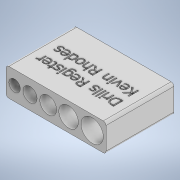
# Autodesk Inventor part: drillRegisterForKevin
Saved by Autodesk Inventor 2022.2 (Build 262287030, 287C)
## iProperties
Created: 2022-02-01
Part Number: drillRegisterForKevin
Material: Generic
Document SubType Name: Modeling
Designer: snobo
Density: 1 g/cm^3
Appearance: Default
Author: snobo
Autodesk Inventor part; units mm, degrees
ref_plane "YZ Plane" through (0, 0, 0) normal (1, 0, 0) x (0, 1, 0)
ref_plane "XZ Plane" through (0, 0, 0) normal (0, 1, 0) x (-1, 0, 0)
ref_plane "XY Plane" through (0, 0, 0) normal (0, 0, 1) x (1, 0, 0)
sketch "Sketch1" plane through (0, 0, 0) normal (0, 0, 1) x (1, 0, 0)
  circle A0 centre (0, 0) radius 13.0175
  circle A1 centre (-27.6225, 0) radius 11.43
  circle A2 centre (-51.4604, 0) radius 9.8425
  circle A3 centre (-72.7329, 0) radius 8.255
  circle A4 centre (-90.8304, 0) radius 6.6675
  line L0 (-90.8304, 0) -> (0, 0) construction
  line L1 (-100.6729, 16.1925) -> (16.1925, 16.1925)
  line L2 (16.1925, 16.1925) -> (16.1925, -16.1925)
  line L3 (16.1925, -16.1925) -> (-100.6729, -16.1925)
  line L4 (-100.6729, -16.1925) -> (-100.6729, 16.1925)
  dimension "d0" = 26.035
  dimension "d1" = 22.86
  dimension "d2" = 3.175
  dimension "d3" = 19.685
  dimension "d4" = 2.5654
  dimension "d5" = 3.175
  dimension "d6" = 16.51
  dimension "d7" = 3.175
  dimension "d8" = 13.335
  dimension "d9" = 3.175
  dimension "d10" = 3.175
  dimension "d11" = 3.175
  dimension "d12" = 3.175
  constraints: 10 end point, 5 centre point, 2 horizontal, 2 parallel, 1 coincident, 1 perpendicular
  measures "d0" diameter of A0
  measures "d1" diameter of A1
  measures "d3" diameter of A2
  measures "d6" diameter of A3
  measures "d8" diameter of A4
  measures "d9" distance edge to line of A0 L2
  measures "d10" distance edge to line of A4 L4
  measures "d11" distance edge to line of A0 L1
  measures "d12" distance edge to line of A0 L3
extrude "Extrusion1" add sketch "Sketch1" against normal blind 76.2
sketch "Sketch2" plane through (0, 0, -76.2) normal (0, 0, -1) x (-1, 0, 0)
  line L0 (-16.1925, -16.1925) -> (-16.1925, 16.1925) projected
  line L1 (-16.1925, 16.1925) -> (100.6729, 16.1925) projected
  line L2 (-16.1925, -16.1925) -> (100.6729, -16.1925)
  line L3 (100.6729, -16.1925) -> (100.6729, 16.1925)
  line L4 (100.6729, 16.1925) -> (-16.1925, 16.1925)
  line L5 (-16.1925, 16.1925) -> (-16.1925, -16.1925)
  point P0 (0, 0)
  constraints: 8 end point, 2 parallel, 1 horizontal, 1 perpendicular
extrude "Extrusion2" add sketch "Sketch2" along normal blind 3.175
fillet "Fillet1" radius 3.175 4 edges at (16.1925, 16.1925, -39.6875) (16.1925, -16.1925, -39.6875) (-100.6729, -16.1925, -39.6875) (-100.6729, 16.1925, -39.6875)
sketch "Sketch3" plane through (-97.4979, 16.1925, 0) normal (0, 1, 0) x (1, 0, 0)
  line L0 (0, 79.375) -> (0, 0) construction
  line L1 (0, 39.6875) -> (110.5154, 39.6875) construction
  line L2 (110.5154, 0) -> (110.5154, 79.375) construction
  spline S0 degree 2 poles (92.8637, 26.3618) (92.8637, 27.9271) (94.1327, 30.4466) (95.1979, 31.1505) knots 0 0 0 1 2 2 2
  spline S1 degree 2 poles (95.1979, 31.1505) (96.0685, 31.697) (97.8562, 32.0675) (99.2456, 32.0675) knots 0 0 0 1 2 2 2
  line L3 (99.2456, 32.0675) -> (101.8762, 32.0675)
  line L4 (101.8762, 32.0675) -> (101.8762, 20.6375)
  line L5 (101.8762, 20.6375) -> (99.2734, 20.6375)
  spline S2 degree 2 poles (99.2734, 20.6375) (97.6617, 20.6375) (95.8277, 21.1192) (95.1793, 21.5452) knots 0 0 0 1 2 2 2
  spline S3 degree 2 poles (95.1793, 21.5452) (94.0771, 22.277) (92.8637, 24.6945) (92.8637, 26.3618) knots 0 0 0 1 2 2 2
  spline S4 degree 2 poles (94.4476, 26.3432) (94.4476, 25.028) (95.3183, 23.1662) (96.1797, 22.6382) knots 0 0 0 1 2 2 2
  spline S5 degree 2 poles (96.1797, 22.6382) (96.791, 22.277) (98.1711, 21.9528) (99.1993, 21.9528) knots 0 0 0 1 2 2 2
  line L6 (99.1993, 21.9528) -> (100.3571, 21.9528)
  line L7 (100.3571, 21.9528) -> (100.3571, 30.7522)
  line L8 (100.3571, 30.7522) -> (99.1993, 30.7522)
  spline S6 degree 2 poles (99.1993, 30.7522) (98.1897, 30.7522) (96.6613, 30.428) (96.0408, 29.9927) knots 0 0 0 1 2 2 2
  spline S7 degree 2 poles (96.0408, 29.9927) (95.2442, 29.4555) (94.4476, 27.677) (94.4476, 26.3432) knots 0 0 0 1 2 2 2
  line L9 (86.7782, 25.0372) -> (86.8523, 25.0372)
  spline S8 degree 2 poles (86.8523, 25.0372) (87.019, 24.9909) (87.3803, 24.9724) (87.6304, 24.9724) knots 0 0 0 1 2 2 2
  spline S9 degree 2 poles (87.6304, 24.9724) (88.2139, 24.9724) (89.3624, 25.4818) (89.8812, 25.982) knots 0 0 0 1 2 2 2
  line L10 (89.8812, 25.982) -> (89.8812, 32.0675)
  line L11 (89.8812, 32.0675) -> (91.3261, 32.0675)
  line L12 (91.3261, 32.0675) -> (91.3261, 23.4904)
  line L13 (91.3261, 23.4904) -> (89.8812, 23.4904)
  line L14 (89.8812, 23.4904) -> (89.8812, 24.7686)
  spline S10 degree 2 poles (89.8812, 24.7686) (89.0938, 24.0646) (87.9175, 23.4904) (87.3617, 23.4904) knots 0 0 0 1 2 2 2
  spline S11 degree 2 poles (87.3617, 23.4904) (87.1394, 23.4904) (86.9171, 23.5089) (86.7782, 23.5367) knots 0 0 0 1 2 2 2
  line L15 (86.7782, 23.5367) -> (86.7782, 25.0372)
  line L16 (84.1847, 32.0675) -> (85.6296, 32.0675)
  line L17 (85.6296, 32.0675) -> (85.6296, 23.4904)
  line L18 (85.6296, 23.4904) -> (84.1847, 23.4904)
  line L19 (84.1847, 23.4904) -> (84.1847, 32.0675)
  line L20 (84.0828, 22.0639) -> (85.7223, 22.0639)
  line L21 (85.7223, 22.0639) -> (85.7223, 20.5634)
  line L22 (85.7223, 20.5634) -> (84.0828, 20.5634)
  line L23 (84.0828, 20.5634) -> (84.0828, 22.0639)
  line L24 (80.5908, 32.0675) -> (82.0358, 32.0675)
  line L25 (82.0358, 32.0675) -> (82.0358, 20.1281)
  line L26 (82.0358, 20.1281) -> (80.5908, 20.1281)
  line L27 (80.5908, 20.1281) -> (80.5908, 32.0675)
  line L28 (76.9969, 32.0675) -> (78.4419, 32.0675)
  line L29 (78.4419, 32.0675) -> (78.4419, 20.1281)
  line L30 (78.4419, 20.1281) -> (76.9969, 20.1281)
  line L31 (76.9969, 20.1281) -> (76.9969, 32.0675)
  spline S12 degree 2 poles (72.5602, 32.2713) (73.4216, 32.2713) (74.9129, 31.8081) (75.4038, 31.5488) knots 0 0 0 1 2 2 2
  line L32 (75.4038, 31.5488) -> (75.4038, 29.9278)
  line L33 (75.4038, 29.9278) -> (75.3297, 29.9278)
  spline S13 degree 2 poles (75.3297, 29.9278) (75.1444, 30.076) (74.6442, 30.428) (74.2274, 30.6225) knots 0 0 0 1 2 2 2
  spline S14 degree 2 poles (74.2274, 30.6225) (73.8662, 30.7985) (72.977, 31.0579) (72.5046, 31.0579) knots 0 0 0 1 2 2 2
  spline S15 degree 2 poles (72.5046, 31.0579) (72.1619, 31.0579) (71.3746, 30.9004) (71.1893, 30.7707) knots 0 0 0 1 2 2 2
  spline S16 degree 2 poles (71.1893, 30.7707) (70.9207, 30.5948) (70.6799, 30.1965) (70.6799, 29.7889) knots 0 0 0 1 2 2 2
  spline S17 degree 2 poles (70.6799, 29.7889) (70.6799, 29.2795) (71.2356, 28.7515) (71.9488, 28.5755) knots 0 0 0 1 2 2 2
  spline S18 degree 2 poles (71.9488, 28.5755) (72.2267, 28.5107) (73.1159, 28.3254) (73.4957, 28.2235) knots 0 0 0 1 2 2 2
  spline S19 degree 2 poles (73.4957, 28.2235) (74.4775, 27.9364) (75.3667, 26.7508) (75.3667, 25.9079) knots 0 0 0 1 2 2 2
  spline S20 degree 2 poles (75.3667, 25.9079) (75.3667, 24.7408) (73.6161, 23.2866) (72.1711, 23.2866) knots 0 0 0 1 2 2 2
  spline S21 degree 2 poles (72.1711, 23.2866) (71.4579, 23.2866) (70.013, 23.6386) (69.522, 23.9072) knots 0 0 0 1 2 2 2
  line L34 (69.522, 23.9072) -> (69.522, 25.454)
  line L35 (69.522, 25.454) -> (69.5961, 25.454)
  spline S22 degree 2 poles (69.5961, 25.454) (70.1519, 25.0094) (71.5042, 24.5) (72.1989, 24.5) knots 0 0 0 1 2 2 2
  spline S23 degree 2 poles (72.1989, 24.5) (72.9121, 24.5) (73.894, 25.1021) (73.894, 25.7041) knots 0 0 0 1 2 2 2
  spline S24 degree 2 poles (73.894, 25.7041) (73.894, 26.2506) (73.3104, 26.7786) (72.6621, 26.9453) knots 0 0 0 1 2 2 2
  spline S25 degree 2 poles (72.6621, 26.9453) (72.3471, 27.0287) (71.5505, 27.1954) (71.1152, 27.2973) knots 0 0 0 1 2 2 2
  spline S26 degree 2 poles (71.1152, 27.2973) (70.1704, 27.5381) (69.2071, 28.6404) (69.2071, 29.5944) knots 0 0 0 1 2 2 2
  spline S27 degree 2 poles (69.2071, 29.5944) (69.2071, 30.1501) (69.6425, 31.132) (70.0685, 31.4932) knots 0 0 0 1 2 2 2
  spline S28 degree 2 poles (70.0685, 31.4932) (70.5224, 31.873) (71.6802, 32.2713) (72.5602, 32.2713) knots 0 0 0 1 2 2 2
  line L36 (53.998, 32.0675) -> (55.9709, 32.0675)
  line L37 (55.9709, 32.0675) -> (59.5833, 27.5196)
  line L38 (59.5833, 27.5196) -> (61.3247, 27.5196)
  line L39 (61.3247, 27.5196) -> (61.3247, 32.0675)
  line L40 (61.3247, 32.0675) -> (62.8437, 32.0675)
  line L41 (62.8437, 32.0675) -> (62.8437, 20.6375)
  line L42 (62.8437, 20.6375) -> (59.8982, 20.6375)
  spline S29 degree 2 poles (59.8982, 20.6375) (58.9164, 20.6375) (57.5919, 20.8505) (56.9898, 21.2396) knots 0 0 0 1 2 2 2
  spline S30 degree 2 poles (56.9898, 21.2396) (56.3877, 21.6286) (55.693, 22.842) (55.693, 23.7405) knots 0 0 0 1 2 2 2
  spline S31 degree 2 poles (55.693, 23.7405) (55.693, 24.9909) (56.9713, 26.686) (58.0643, 27.0935) knots 0 0 0 1 2 2 2
  line L43 (58.0643, 27.0935) -> (53.998, 32.0675)
  spline S32 degree 2 poles (57.2769, 23.8609) (57.2769, 23.3607) (57.6289, 22.5919) (57.9994, 22.3418) knots 0 0 0 1 2 2 2
  spline S33 degree 2 poles (57.9994, 22.3418) (58.3236, 22.1288) (59.185, 21.9528) (59.8149, 21.9528) knots 0 0 0 1 2 2 2
  line L44 (59.8149, 21.9528) -> (61.3247, 21.9528)
  line L45 (61.3247, 21.9528) -> (61.3247, 26.2506)
  line L46 (61.3247, 26.2506) -> (59.9909, 26.2506)
  spline S34 degree 2 poles (59.9909, 26.2506) (59.3332, 26.2506) (58.2866, 26.019) (57.9253, 25.6578) knots 0 0 0 1 2 2 2
  spline S35 degree 2 poles (57.9253, 25.6578) (57.5919, 25.3429) (57.2769, 24.4537) (57.2769, 23.8609) knots 0 0 0 1 2 2 2
  spline S36 degree 2 poles (49.4779, 32.262) (51.5342, 32.262) (53.7942, 29.9556) (53.7942, 27.8252) knots 0 0 0 1 2 2 2
  spline S37 degree 2 poles (53.7942, 27.8252) (53.7942, 25.7319) (51.599, 23.2495) (49.8298, 23.2495) knots 0 0 0 1 2 2 2
  spline S38 degree 2 poles (49.8298, 23.2495) (49.0333, 23.2495) (47.8013, 23.7127) (47.3475, 24.2036) knots 0 0 0 1 2 2 2
  spline S39 degree 2 poles (47.3475, 24.2036) (46.8843, 24.6945) (46.3934, 26.1117) (46.3934, 27.1398) knots 0 0 0 1 2 2 2
  line L47 (46.3934, 27.1398) -> (46.3934, 27.9271)
  line L48 (46.3934, 27.9271) -> (52.3307, 27.9271)
  spline S40 degree 2 poles (52.3307, 27.9271) (52.3307, 29.4184) (50.8302, 31.0023) (49.4964, 31.0023) knots 0 0 0 1 2 2 2
  spline S41 degree 2 poles (49.4964, 31.0023) (49.024, 31.0023) (48.107, 30.7893) (47.7365, 30.6225) knots 0 0 0 1 2 2 2
  spline S42 degree 2 poles (47.7365, 30.6225) (47.3475, 30.4373) (46.8102, 30.1131) (46.6343, 29.9649) knots 0 0 0 1 2 2 2
  line L49 (46.6343, 29.9649) -> (46.5509, 29.9649)
  line L50 (46.5509, 29.9649) -> (46.5509, 31.5395)
  spline S43 degree 2 poles (46.5509, 31.5395) (46.801, 31.6414) (47.5605, 31.9378) (47.8569, 32.0212) knots 0 0 0 1 2 2 2
  spline S44 degree 2 poles (47.8569, 32.0212) (48.2737, 32.1416) (48.9592, 32.262) (49.4779, 32.262) knots 0 0 0 1 2 2 2
  spline S45 degree 2 poles (47.8013, 26.8249) (47.8199, 26.2413) (48.0607, 25.3892) (48.2923, 25.1021) knots 0 0 0 1 2 2 2
  spline S46 degree 2 poles (48.2923, 25.1021) (48.5423, 24.7779) (49.3297, 24.4351) (49.9132, 24.4351) knots 0 0 0 1 2 2 2
  spline S47 degree 2 poles (49.9132, 24.4351) (50.4875, 24.4351) (51.2933, 24.7779) (51.6268, 25.1113) knots 0 0 0 1 2 2 2
  spline S48 degree 2 poles (51.6268, 25.1113) (51.951, 25.454) (52.2844, 26.2784) (52.3307, 26.8249) knots 0 0 0 1 2 2 2
  line L51 (52.3307, 26.8249) -> (47.8013, 26.8249)
  spline S49 degree 2 poles (44.6243, 33.4384) (44.4761, 33.5032) (43.9111, 33.707) (43.5498, 33.7903) knots 0 0 0 1 2 2 2
  spline S50 degree 2 poles (43.5498, 33.7903) (43.1515, 33.8922) (42.4754, 34.0126) (42.0771, 34.0126) knots 0 0 0 1 2 2 2
  spline S51 degree 2 poles (42.0771, 34.0126) (41.4102, 34.0126) (40.4839, 33.6607) (40.2246, 33.3457) knots 0 0 0 1 2 2 2
  spline S52 degree 2 poles (40.2246, 33.3457) (39.9745, 33.0308) (39.78, 32.2064) (39.78, 31.6785) knots 0 0 0 1 2 2 2
  line L52 (39.78, 31.6785) -> (39.78, 30.9282)
  spline S53 degree 2 poles (39.78, 30.9282) (40.3635, 31.4376) (41.4843, 31.9193) (42.3272, 31.9193) knots 0 0 0 1 2 2 2
  spline S54 degree 2 poles (42.3272, 31.9193) (43.7907, 31.9193) (45.5227, 29.7426) (45.5227, 27.6956) knots 0 0 0 1 2 2 2
  spline S55 degree 2 poles (45.5227, 27.6956) (45.5227, 26.6304) (44.9207, 24.9816) (44.4205, 24.3981) knots 0 0 0 1 2 2 2
  spline S56 degree 2 poles (44.4205, 24.3981) (43.9389, 23.8516) (42.6143, 23.2495) (41.9104, 23.2495) knots 0 0 0 1 2 2 2
  spline S57 degree 2 poles (41.9104, 23.2495) (41.2434, 23.2495) (40.2709, 23.5645) (39.78, 23.8516) knots 0 0 0 1 2 2 2
  line L53 (39.78, 23.8516) -> (39.6966, 23.4904)
  line L54 (39.6966, 23.4904) -> (38.335, 23.4904)
  line L55 (38.335, 23.4904) -> (38.335, 31.0857)
  spline S58 degree 2 poles (38.335, 31.0857) (38.335, 33.2716) (40.2338, 35.3094) (42.1882, 35.3094) knots 0 0 0 1 2 2 2
  spline S59 degree 2 poles (42.1882, 35.3094) (42.8181, 35.3094) (44.1334, 35.1056) (44.6984, 34.9389) knots 0 0 0 1 2 2 2
  line L56 (44.6984, 34.9389) -> (44.6984, 33.4384)
  line L57 (44.6984, 33.4384) -> (44.6243, 33.4384)
  line L58 (39.78, 29.7426) -> (39.78, 25.028)
  spline S60 degree 2 poles (39.78, 25.028) (40.3172, 24.7686) (41.2249, 24.5463) (41.6788, 24.5463) knots 0 0 0 1 2 2 2
  spline S61 degree 2 poles (41.6788, 24.5463) (42.7718, 24.5463) (44.0315, 26.158) (44.0315, 27.6678) knots 0 0 0 1 2 2 2
  spline S62 degree 2 poles (44.0315, 27.6678) (44.0315, 29.0942) (43.0774, 30.5855) (42.003, 30.5855) knots 0 0 0 1 2 2 2
  spline S63 degree 2 poles (42.003, 30.5855) (41.438, 30.5855) (40.2524, 30.1409) (39.78, 29.7426) knots 0 0 0 1 2 2 2
  line L59 (34.7689, 32.0675) -> (36.2139, 32.0675)
  line L60 (36.2139, 32.0675) -> (36.2139, 23.4904)
  line L61 (36.2139, 23.4904) -> (34.7689, 23.4904)
  line L62 (34.7689, 23.4904) -> (34.7689, 32.0675)
  line L63 (34.667, 22.0639) -> (36.3065, 22.0639)
  line L64 (36.3065, 22.0639) -> (36.3065, 20.5634)
  line L65 (36.3065, 20.5634) -> (34.667, 20.5634)
  line L66 (34.667, 20.5634) -> (34.667, 22.0639)
  spline S64 degree 2 poles (30.3322, 32.2713) (31.1936, 32.2713) (32.6848, 31.8081) (33.1758, 31.5488) knots 0 0 0 1 2 2 2
  line L67 (33.1758, 31.5488) -> (33.1758, 29.9278)
  line L68 (33.1758, 29.9278) -> (33.1017, 29.9278)
  spline S65 degree 2 poles (33.1017, 29.9278) (32.9164, 30.076) (32.4162, 30.428) (31.9994, 30.6225) knots 0 0 0 1 2 2 2
  spline S66 degree 2 poles (31.9994, 30.6225) (31.6382, 30.7985) (30.749, 31.0579) (30.2766, 31.0579) knots 0 0 0 1 2 2 2
  spline S67 degree 2 poles (30.2766, 31.0579) (29.9339, 31.0579) (29.1465, 30.9004) (28.9613, 30.7707) knots 0 0 0 1 2 2 2
  spline S68 degree 2 poles (28.9613, 30.7707) (28.6927, 30.5948) (28.4519, 30.1965) (28.4519, 29.7889) knots 0 0 0 1 2 2 2
  spline S69 degree 2 poles (28.4519, 29.7889) (28.4519, 29.2795) (29.0076, 28.7515) (29.7208, 28.5755) knots 0 0 0 1 2 2 2
  spline S70 degree 2 poles (29.7208, 28.5755) (29.9987, 28.5107) (30.8879, 28.3254) (31.2677, 28.2235) knots 0 0 0 1 2 2 2
  spline S71 degree 2 poles (31.2677, 28.2235) (32.2495, 27.9364) (33.1387, 26.7508) (33.1387, 25.9079) knots 0 0 0 1 2 2 2
  spline S72 degree 2 poles (33.1387, 25.9079) (33.1387, 24.7408) (31.3881, 23.2866) (29.9431, 23.2866) knots 0 0 0 1 2 2 2
  spline S73 degree 2 poles (29.9431, 23.2866) (29.2299, 23.2866) (27.7849, 23.6386) (27.294, 23.9072) knots 0 0 0 1 2 2 2
  line L69 (27.294, 23.9072) -> (27.294, 25.454)
  line L70 (27.294, 25.454) -> (27.3681, 25.454)
  spline S74 degree 2 poles (27.3681, 25.454) (27.9239, 25.0094) (29.2762, 24.5) (29.9709, 24.5) knots 0 0 0 1 2 2 2
  spline S75 degree 2 poles (29.9709, 24.5) (30.6841, 24.5) (31.666, 25.1021) (31.666, 25.7041) knots 0 0 0 1 2 2 2
  spline S76 degree 2 poles (31.666, 25.7041) (31.666, 26.2506) (31.0824, 26.7786) (30.434, 26.9453) knots 0 0 0 1 2 2 2
  spline S77 degree 2 poles (30.434, 26.9453) (30.1191, 27.0287) (29.3225, 27.1954) (28.8872, 27.2973) knots 0 0 0 1 2 2 2
  spline S78 degree 2 poles (28.8872, 27.2973) (27.9424, 27.5381) (26.9791, 28.6404) (26.9791, 29.5944) knots 0 0 0 1 2 2 2
  spline S79 degree 2 poles (26.9791, 29.5944) (26.9791, 30.1501) (27.4144, 31.132) (27.8405, 31.4932) knots 0 0 0 1 2 2 2
  spline S80 degree 2 poles (27.8405, 31.4932) (28.2944, 31.873) (29.4522, 32.2713) (30.3322, 32.2713) knots 0 0 0 1 2 2 2
  spline S81 degree 2 poles (23.0425, 32.2342) (24.2189, 32.2342) (25.5434, 30.8912) (25.5434, 29.4369) knots 0 0 0 1 2 2 2
  line L71 (25.5434, 29.4369) -> (25.5434, 24.6852)
  line L72 (25.5434, 24.6852) -> (26.516, 24.6852)
  line L73 (26.516, 24.6852) -> (26.516, 23.4904)
  line L74 (26.516, 23.4904) -> (25.5434, 23.4904)
  line L75 (25.5434, 23.4904) -> (25.5434, 21.0265)
  line L76 (25.5434, 21.0265) -> (24.0984, 21.0265)
  line L77 (24.0984, 21.0265) -> (24.0984, 23.4904)
  line L78 (24.0984, 23.4904) -> (21.4401, 23.4904)
  line L79 (21.4401, 23.4904) -> (21.4401, 24.6852)
  line L80 (21.4401, 24.6852) -> (24.0984, 24.6852)
  line L81 (24.0984, 24.6852) -> (24.0984, 28.77)
  spline S82 degree 2 poles (24.0984, 28.77) (24.0984, 29.4184) (24.0521, 30.1316) (23.8947, 30.4373) knots 0 0 0 1 2 2 2
  spline S83 degree 2 poles (23.8947, 30.4373) (23.765, 30.7059) (23.1815, 30.9745) (22.6813, 30.9745) knots 0 0 0 1 2 2 2
  spline S84 degree 2 poles (22.6813, 30.9745) (22.3293, 30.9745) (21.6717, 30.7615) (21.5235, 30.6966) knots 0 0 0 1 2 2 2
  line L82 (21.5235, 30.6966) -> (21.4401, 30.6966)
  line L83 (21.4401, 30.6966) -> (21.4401, 31.9934)
  spline S85 degree 2 poles (21.4401, 31.9934) (21.8476, 32.1046) (22.6813, 32.2342) (23.0425, 32.2342) knots 0 0 0 1 2 2 2
  spline S86 degree 2 poles (16.6513, 32.262) (18.7076, 32.262) (20.9677, 29.9556) (20.9677, 27.8252) knots 0 0 0 1 2 2 2
  spline S87 degree 2 poles (20.9677, 27.8252) (20.9677, 25.7319) (18.7725, 23.2495) (17.0033, 23.2495) knots 0 0 0 1 2 2 2
  spline S88 degree 2 poles (17.0033, 23.2495) (16.2067, 23.2495) (14.9748, 23.7127) (14.521, 24.2036) knots 0 0 0 1 2 2 2
  spline S89 degree 2 poles (14.521, 24.2036) (14.0578, 24.6945) (13.5669, 26.1117) (13.5669, 27.1398) knots 0 0 0 1 2 2 2
  line L84 (13.5669, 27.1398) -> (13.5669, 27.9271)
  line L85 (13.5669, 27.9271) -> (19.5042, 27.9271)
  spline S90 degree 2 poles (19.5042, 27.9271) (19.5042, 29.4184) (18.0037, 31.0023) (16.6699, 31.0023) knots 0 0 0 1 2 2 2
  spline S91 degree 2 poles (16.6699, 31.0023) (16.1975, 31.0023) (15.2805, 30.7893) (14.91, 30.6225) knots 0 0 0 1 2 2 2
  spline S92 degree 2 poles (14.91, 30.6225) (14.521, 30.4373) (13.9837, 30.1131) (13.8077, 29.9649) knots 0 0 0 1 2 2 2
  line L86 (13.8077, 29.9649) -> (13.7244, 29.9649)
  line L87 (13.7244, 29.9649) -> (13.7244, 31.5395)
  spline S93 degree 2 poles (13.7244, 31.5395) (13.9745, 31.6414) (14.734, 31.9378) (15.0304, 32.0212) knots 0 0 0 1 2 2 2
  spline S94 degree 2 poles (15.0304, 32.0212) (15.4472, 32.1416) (16.1326, 32.262) (16.6513, 32.262) knots 0 0 0 1 2 2 2
  spline S95 degree 2 poles (14.9748, 26.8249) (14.9933, 26.2413) (15.2342, 25.3892) (15.4657, 25.1021) knots 0 0 0 1 2 2 2
  spline S96 degree 2 poles (15.4657, 25.1021) (15.7158, 24.7779) (16.5031, 24.4351) (17.0867, 24.4351) knots 0 0 0 1 2 2 2
  spline S97 degree 2 poles (17.0867, 24.4351) (17.661, 24.4351) (18.4668, 24.7779) (18.8003, 25.1113) knots 0 0 0 1 2 2 2
  spline S98 degree 2 poles (18.8003, 25.1113) (19.1245, 25.454) (19.4579, 26.2784) (19.5042, 26.8249) knots 0 0 0 1 2 2 2
  line L88 (19.5042, 26.8249) -> (14.9748, 26.8249)
  line L89 (7.5555, 25.0372) -> (7.6296, 25.0372)
  spline S99 degree 2 poles (7.6296, 25.0372) (7.7963, 24.9909) (8.1576, 24.9724) (8.4077, 24.9724) knots 0 0 0 1 2 2 2
  spline S100 degree 2 poles (8.4077, 24.9724) (8.9912, 24.9724) (10.1398, 25.4818) (10.6585, 25.982) knots 0 0 0 1 2 2 2
  line L90 (10.6585, 25.982) -> (10.6585, 32.0675)
  line L91 (10.6585, 32.0675) -> (12.1034, 32.0675)
  line L92 (12.1034, 32.0675) -> (12.1034, 23.4904)
  line L93 (12.1034, 23.4904) -> (10.6585, 23.4904)
  line L94 (10.6585, 23.4904) -> (10.6585, 24.7686)
  spline S101 degree 2 poles (10.6585, 24.7686) (9.8712, 24.0646) (8.6948, 23.4904) (8.1391, 23.4904) knots 0 0 0 1 2 2 2
  spline S102 degree 2 poles (8.1391, 23.4904) (7.9168, 23.4904) (7.6945, 23.5089) (7.5555, 23.5367) knots 0 0 0 1 2 2 2
  line L95 (7.5555, 23.5367) -> (7.5555, 25.0372)
  line L96 (92.5766, 51.2112) -> (94.5495, 51.2112)
  line L97 (94.5495, 51.2112) -> (98.7269, 45.8944)
  line L98 (98.7269, 45.8944) -> (99.3938, 46.6447)
  line L99 (99.3938, 46.6447) -> (99.3938, 51.2112)
  line L100 (99.3938, 51.2112) -> (100.9129, 51.2112)
  line L101 (100.9129, 51.2112) -> (100.9129, 39.7812)
  line L102 (100.9129, 39.7812) -> (99.3938, 39.7812)
  line L103 (99.3938, 39.7812) -> (99.3938, 45.033)
  line L104 (99.3938, 45.033) -> (94.7069, 39.7812)
  line L105 (94.7069, 39.7812) -> (92.8544, 39.7812)
  line L106 (92.8544, 39.7812) -> (97.5876, 44.8848)
  line L107 (97.5876, 44.8848) -> (92.5766, 51.2112)
  spline S103 degree 2 poles (88.0564, 51.4057) (90.1127, 51.4057) (92.3728, 49.0993) (92.3728, 46.9689) knots 0 0 0 1 2 2 2
  spline S104 degree 2 poles (92.3728, 46.9689) (92.3728, 44.8756) (90.1776, 42.3932) (88.4084, 42.3932) knots 0 0 0 1 2 2 2
  spline S105 degree 2 poles (88.4084, 42.3932) (87.6118, 42.3932) (86.3799, 42.8563) (85.926, 43.3472) knots 0 0 0 1 2 2 2
  spline S106 degree 2 poles (85.926, 43.3472) (85.4629, 43.8382) (84.972, 45.2553) (84.972, 46.2835) knots 0 0 0 1 2 2 2
  line L108 (84.972, 46.2835) -> (84.972, 47.0708)
  line L109 (84.972, 47.0708) -> (90.9093, 47.0708)
  spline S107 degree 2 poles (90.9093, 47.0708) (90.9093, 48.5621) (89.4088, 50.146) (88.075, 50.146) knots 0 0 0 1 2 2 2
  spline S108 degree 2 poles (88.075, 50.146) (87.6026, 50.146) (86.6856, 49.9329) (86.3151, 49.7662) knots 0 0 0 1 2 2 2
  spline S109 degree 2 poles (86.3151, 49.7662) (85.926, 49.5809) (85.3888, 49.2568) (85.2128, 49.1085) knots 0 0 0 1 2 2 2
  line L110 (85.2128, 49.1085) -> (85.1295, 49.1085)
  line L111 (85.1295, 49.1085) -> (85.1295, 50.6832)
  spline S110 degree 2 poles (85.1295, 50.6832) (85.3795, 50.7851) (86.1391, 51.0815) (86.4355, 51.1648) knots 0 0 0 1 2 2 2
  spline S111 degree 2 poles (86.4355, 51.1648) (86.8523, 51.2853) (87.5377, 51.4057) (88.0564, 51.4057) knots 0 0 0 1 2 2 2
  spline S112 degree 2 poles (86.3799, 45.9685) (86.3984, 45.385) (86.6393, 44.5328) (86.8708, 44.2457) knots 0 0 0 1 2 2 2
  spline S113 degree 2 poles (86.8708, 44.2457) (87.1209, 43.9215) (87.9082, 43.5788) (88.4918, 43.5788) knots 0 0 0 1 2 2 2
  spline S114 degree 2 poles (88.4918, 43.5788) (89.066, 43.5788) (89.8719, 43.9215) (90.2053, 44.255) knots 0 0 0 1 2 2 2
  spline S115 degree 2 poles (90.2053, 44.255) (90.5295, 44.5977) (90.863, 45.4221) (90.9093, 45.9685) knots 0 0 0 1 2 2 2
  line L112 (90.9093, 45.9685) -> (86.3799, 45.9685)
  line L113 (76.7746, 42.634) -> (80.0073, 51.2112)
  line L114 (80.0073, 51.2112) -> (81.304, 51.2112)
  line L115 (81.304, 51.2112) -> (84.5089, 42.634)
  line L116 (84.5089, 42.634) -> (82.9435, 42.634)
  line L117 (82.9435, 42.634) -> (80.6001, 49.2382)
  line L118 (80.6001, 49.2382) -> (78.2752, 42.634)
  line L119 (78.2752, 42.634) -> (76.7746, 42.634)
  line L120 (74.2089, 51.2112) -> (75.6539, 51.2112)
  line L121 (75.6539, 51.2112) -> (75.6539, 42.634)
  line L122 (75.6539, 42.634) -> (74.2089, 42.634)
  line L123 (74.2089, 42.634) -> (74.2089, 51.2112)
  line L124 (74.107, 41.2076) -> (75.7465, 41.2076)
  line L125 (75.7465, 41.2076) -> (75.7465, 39.707)
  line L126 (75.7465, 39.707) -> (74.107, 39.707)
  line L127 (74.107, 39.707) -> (74.107, 41.2076)
  line L128 (65.3539, 51.2112) -> (66.7989, 51.2112)
  line L129 (66.7989, 51.2112) -> (66.7989, 46.3205)
  spline S116 degree 2 poles (66.7989, 46.3205) (66.7989, 45.7277) (66.91, 44.7088) (67.0767, 44.4032) knots 0 0 0 1 2 2 2
  spline S117 degree 2 poles (67.0767, 44.4032) (67.2527, 44.079) (67.8826, 43.7641) (68.4198, 43.7641) knots 0 0 0 1 2 2 2
  spline S118 degree 2 poles (68.4198, 43.7641) (68.957, 43.7641) (70.0963, 44.3383) (70.6428, 44.8015) knots 0 0 0 1 2 2 2
  line L130 (70.6428, 44.8015) -> (70.6428, 51.2112)
  line L131 (70.6428, 51.2112) -> (72.0878, 51.2112)
  line L132 (72.0878, 51.2112) -> (72.0878, 42.634)
  line L133 (72.0878, 42.634) -> (70.6428, 42.634)
  line L134 (70.6428, 42.634) -> (70.6428, 43.5881)
  spline S119 degree 2 poles (70.6428, 43.5881) (69.9944, 43.0045) (68.744, 42.3932) (68.04, 42.3932) knots 0 0 0 1 2 2 2
  spline S120 degree 2 poles (68.04, 42.3932) (66.7803, 42.3932) (65.3539, 44.0605) (65.3539, 45.6444) knots 0 0 0 1 2 2 2
  line L135 (65.3539, 45.6444) -> (65.3539, 51.2112)
  line L136 (49.4593, 51.2112) -> (51.4323, 51.2112)
  line L137 (51.4323, 51.2112) -> (55.0447, 46.6632)
  line L138 (55.0447, 46.6632) -> (56.786, 46.6632)
  line L139 (56.786, 46.6632) -> (56.786, 51.2112)
  line L140 (56.786, 51.2112) -> (58.3051, 51.2112)
  line L141 (58.3051, 51.2112) -> (58.3051, 39.7812)
  line L142 (58.3051, 39.7812) -> (55.3596, 39.7812)
  spline S121 degree 2 poles (55.3596, 39.7812) (54.3778, 39.7812) (53.0532, 39.9942) (52.4511, 40.3832) knots 0 0 0 1 2 2 2
  spline S122 degree 2 poles (52.4511, 40.3832) (51.8491, 40.7722) (51.1544, 41.9856) (51.1544, 42.8841) knots 0 0 0 1 2 2 2
  spline S123 degree 2 poles (51.1544, 42.8841) (51.1544, 44.1346) (52.4326, 45.8296) (53.5256, 46.2372) knots 0 0 0 1 2 2 2
  line L143 (53.5256, 46.2372) -> (49.4593, 51.2112)
  spline S124 degree 2 poles (52.7383, 43.0045) (52.7383, 42.5043) (53.0903, 41.7356) (53.4608, 41.4855) knots 0 0 0 1 2 2 2
  spline S125 degree 2 poles (53.4608, 41.4855) (53.785, 41.2724) (54.6464, 41.0964) (55.2762, 41.0964) knots 0 0 0 1 2 2 2
  line L144 (55.2762, 41.0964) -> (56.786, 41.0964)
  line L145 (56.786, 41.0964) -> (56.786, 45.3943)
  line L146 (56.786, 45.3943) -> (55.4522, 45.3943)
  spline S126 degree 2 poles (55.4522, 45.3943) (54.7946, 45.3943) (53.7479, 45.1627) (53.3867, 44.8015) knots 0 0 0 1 2 2 2
  spline S127 degree 2 poles (53.3867, 44.8015) (53.0532, 44.4865) (52.7383, 43.5973) (52.7383, 43.0045) knots 0 0 0 1 2 2 2
  line L147 (41.9289, 51.2112) -> (43.3738, 51.2112)
  line L148 (43.3738, 51.2112) -> (43.3738, 46.3205)
  spline S128 degree 2 poles (43.3738, 46.3205) (43.3738, 45.7277) (43.485, 44.7088) (43.6517, 44.4032) knots 0 0 0 1 2 2 2
  spline S129 degree 2 poles (43.6517, 44.4032) (43.8277, 44.079) (44.4576, 43.7641) (44.9948, 43.7641) knots 0 0 0 1 2 2 2
  spline S130 degree 2 poles (44.9948, 43.7641) (45.532, 43.7641) (46.6713, 44.3383) (47.2178, 44.8015) knots 0 0 0 1 2 2 2
  line L149 (47.2178, 44.8015) -> (47.2178, 51.2112)
  line L150 (47.2178, 51.2112) -> (48.6628, 51.2112)
  line L151 (48.6628, 51.2112) -> (48.6628, 39.2717)
  line L152 (48.6628, 39.2717) -> (47.2178, 39.2717)
  line L153 (47.2178, 39.2717) -> (47.2178, 43.5881)
  spline S131 degree 2 poles (47.2178, 43.5881) (46.5694, 43.0045) (45.319, 42.3932) (44.615, 42.3932) knots 0 0 0 1 2 2 2
  spline S132 degree 2 poles (44.615, 42.3932) (43.3553, 42.3932) (41.9289, 44.0605) (41.9289, 45.6444) knots 0 0 0 1 2 2 2
  line L154 (41.9289, 45.6444) -> (41.9289, 51.2112)
  spline S133 degree 2 poles (32.8516, 46.9226) (32.8516, 49.09) (34.9356, 51.452) (36.677, 51.452) knots 0 0 0 1 2 2 2
  spline S134 degree 2 poles (36.677, 51.452) (38.4647, 51.452) (40.5117, 49.0159) (40.5117, 46.9226) knots 0 0 0 1 2 2 2
  spline S135 degree 2 poles (40.5117, 46.9226) (40.5117, 44.7737) (38.3998, 42.3932) (36.677, 42.3932) knots 0 0 0 1 2 2 2
  spline S136 degree 2 poles (36.677, 42.3932) (34.9356, 42.3932) (32.8516, 44.7644) (32.8516, 46.9226) knots 0 0 0 1 2 2 2
  spline S137 degree 2 poles (34.3428, 46.9226) (34.3428, 45.2553) (35.5562, 43.6344) (36.677, 43.6344) knots 0 0 0 1 2 2 2
  spline S138 degree 2 poles (36.677, 43.6344) (37.7978, 43.6344) (39.0204, 45.2553) (39.0204, 46.9226) knots 0 0 0 1 2 2 2
  spline S139 degree 2 poles (39.0204, 46.9226) (39.0204, 48.5435) (37.7978, 50.2108) (36.677, 50.2108) knots 0 0 0 1 2 2 2
  spline S140 degree 2 poles (36.677, 50.2108) (35.5655, 50.2108) (34.3428, 48.5713) (34.3428, 46.9226) knots 0 0 0 1 2 2 2
  line L155 (24.7746, 51.2112) -> (26.2196, 51.2112)
  line L156 (26.2196, 51.2112) -> (26.2196, 50.3405)
  spline S141 degree 2 poles (26.2196, 50.3405) (26.553, 50.6183) (27.0439, 50.9888) (27.3774, 51.1463) knots 0 0 0 1 2 2 2
  spline S142 degree 2 poles (27.3774, 51.1463) (27.6831, 51.2945) (28.3407, 51.452) (28.776, 51.452) knots 0 0 0 1 2 2 2
  spline S143 degree 2 poles (28.776, 51.452) (29.48, 51.452) (30.6656, 50.8684) (31.0824, 50.3034) knots 0 0 0 1 2 2 2
  spline S144 degree 2 poles (31.0824, 50.3034) (31.4992, 49.7384) (31.9624, 48.0711) (31.9624, 46.9874) knots 0 0 0 1 2 2 2
  spline S145 degree 2 poles (31.9624, 46.9874) (31.9624, 45.8574) (31.3788, 44.2087) (30.8694, 43.5881) knots 0 0 0 1 2 2 2
  spline S146 degree 2 poles (30.8694, 43.5881) (30.397, 43.0323) (29.0724, 42.3932) (28.3407, 42.3932) knots 0 0 0 1 2 2 2
  spline S147 degree 2 poles (28.3407, 42.3932) (27.7016, 42.3932) (26.7475, 42.6803) (26.2196, 42.9767) knots 0 0 0 1 2 2 2
  line L157 (26.2196, 42.9767) -> (26.2196, 39.2717)
  line L158 (26.2196, 39.2717) -> (24.7746, 39.2717)
  line L159 (24.7746, 39.2717) -> (24.7746, 51.2112)
  line L160 (26.2196, 49.1271) -> (26.2196, 44.1716)
  spline S148 degree 2 poles (26.2196, 44.1716) (26.7568, 43.9123) (27.609, 43.7177) (28.0999, 43.7177) knots 0 0 0 1 2 2 2
  spline S149 degree 2 poles (28.0999, 43.7177) (29.2114, 43.7177) (30.4711, 45.385) (30.4711, 46.9596) knots 0 0 0 1 2 2 2
  spline S150 degree 2 poles (30.4711, 46.9596) (30.4711, 48.4787) (29.5078, 50.0811) (28.4426, 50.0811) knots 0 0 0 1 2 2 2
  spline S151 degree 2 poles (28.4426, 50.0811) (27.8776, 50.0811) (26.729, 49.5624) (26.2196, 49.1271) knots 0 0 0 1 2 2 2
  spline S152 degree 2 poles (18.9577, 51.4057) (21.014, 51.4057) (23.2741, 49.0993) (23.2741, 46.9689) knots 0 0 0 1 2 2 2
  spline S153 degree 2 poles (23.2741, 46.9689) (23.2741, 44.8756) (21.0789, 42.3932) (19.3097, 42.3932) knots 0 0 0 1 2 2 2
  spline S154 degree 2 poles (19.3097, 42.3932) (18.5131, 42.3932) (17.2812, 42.8563) (16.8273, 43.3472) knots 0 0 0 1 2 2 2
  spline S155 degree 2 poles (16.8273, 43.3472) (16.3642, 43.8382) (15.8733, 45.2553) (15.8733, 46.2835) knots 0 0 0 1 2 2 2
  line L161 (15.8733, 46.2835) -> (15.8733, 47.0708)
  line L162 (15.8733, 47.0708) -> (21.8106, 47.0708)
  spline S156 degree 2 poles (21.8106, 47.0708) (21.8106, 48.5621) (20.3101, 50.146) (18.9763, 50.146) knots 0 0 0 1 2 2 2
  spline S157 degree 2 poles (18.9763, 50.146) (18.5039, 50.146) (17.5869, 49.9329) (17.2164, 49.7662) knots 0 0 0 1 2 2 2
  spline S158 degree 2 poles (17.2164, 49.7662) (16.8273, 49.5809) (16.2901, 49.2568) (16.1141, 49.1085) knots 0 0 0 1 2 2 2
  line L163 (16.1141, 49.1085) -> (16.0308, 49.1085)
  line L164 (16.0308, 49.1085) -> (16.0308, 50.6832)
  spline S159 degree 2 poles (16.0308, 50.6832) (16.2808, 50.7851) (17.0404, 51.0815) (17.3368, 51.1648) knots 0 0 0 1 2 2 2
  spline S160 degree 2 poles (17.3368, 51.1648) (17.7536, 51.2853) (18.439, 51.4057) (18.9577, 51.4057) knots 0 0 0 1 2 2 2
  spline S161 degree 2 poles (17.2812, 45.9685) (17.2997, 45.385) (17.5406, 44.5328) (17.7721, 44.2457) knots 0 0 0 1 2 2 2
  spline S162 degree 2 poles (17.7721, 44.2457) (18.0222, 43.9215) (18.8095, 43.5788) (19.3931, 43.5788) knots 0 0 0 1 2 2 2
  spline S163 degree 2 poles (19.3931, 43.5788) (19.9673, 43.5788) (20.7732, 43.9215) (21.1066, 44.255) knots 0 0 0 1 2 2 2
  spline S164 degree 2 poles (21.1066, 44.255) (21.4308, 44.5977) (21.7643, 45.4221) (21.8106, 45.9685) knots 0 0 0 1 2 2 2
  line L165 (21.8106, 45.9685) -> (17.2812, 45.9685)
  spline S165 degree 2 poles (12.0942, 51.4149) (12.9556, 51.4149) (14.4469, 50.9518) (14.9378, 50.6924) knots 0 0 0 1 2 2 2
  line L166 (14.9378, 50.6924) -> (14.9378, 49.0715)
  line L167 (14.9378, 49.0715) -> (14.8637, 49.0715)
  spline S166 degree 2 poles (14.8637, 49.0715) (14.6784, 49.2197) (14.1782, 49.5717) (13.7614, 49.7662) knots 0 0 0 1 2 2 2
  spline S167 degree 2 poles (13.7614, 49.7662) (13.4002, 49.9422) (12.511, 50.2015) (12.0386, 50.2015) knots 0 0 0 1 2 2 2
  spline S168 degree 2 poles (12.0386, 50.2015) (11.6959, 50.2015) (10.9086, 50.0441) (10.7233, 49.9144) knots 0 0 0 1 2 2 2
  spline S169 degree 2 poles (10.7233, 49.9144) (10.4547, 49.7384) (10.2139, 49.3401) (10.2139, 48.9326) knots 0 0 0 1 2 2 2
  spline S170 degree 2 poles (10.2139, 48.9326) (10.2139, 48.4231) (10.7696, 47.8952) (11.4828, 47.7192) knots 0 0 0 1 2 2 2
  spline S171 degree 2 poles (11.4828, 47.7192) (11.7607, 47.6543) (12.6499, 47.4691) (13.0297, 47.3672) knots 0 0 0 1 2 2 2
  spline S172 degree 2 poles (13.0297, 47.3672) (14.0115, 47.08) (14.9007, 45.8944) (14.9007, 45.0515) knots 0 0 0 1 2 2 2
  spline S173 degree 2 poles (14.9007, 45.0515) (14.9007, 43.8845) (13.1501, 42.4302) (11.7051, 42.4302) knots 0 0 0 1 2 2 2
  spline S174 degree 2 poles (11.7051, 42.4302) (10.9919, 42.4302) (9.547, 42.7822) (9.056, 43.0508) knots 0 0 0 1 2 2 2
  line L168 (9.056, 43.0508) -> (9.056, 44.5977)
  line L169 (9.056, 44.5977) -> (9.1302, 44.5977)
  spline S175 degree 2 poles (9.1302, 44.5977) (9.6859, 44.1531) (11.0382, 43.6436) (11.7329, 43.6436) knots 0 0 0 1 2 2 2
  spline S176 degree 2 poles (11.7329, 43.6436) (12.4461, 43.6436) (13.428, 44.2457) (13.428, 44.8478) knots 0 0 0 1 2 2 2
  spline S177 degree 2 poles (13.428, 44.8478) (13.428, 45.3943) (12.8444, 45.9222) (12.1961, 46.089) knots 0 0 0 1 2 2 2
  spline S178 degree 2 poles (12.1961, 46.089) (11.8811, 46.1723) (11.0846, 46.339) (10.6492, 46.4409) knots 0 0 0 1 2 2 2
  spline S179 degree 2 poles (10.6492, 46.4409) (9.7044, 46.6818) (8.7411, 47.784) (8.7411, 48.738) knots 0 0 0 1 2 2 2
  spline S180 degree 2 poles (8.7411, 48.738) (8.7411, 49.2938) (9.1765, 50.2756) (9.6025, 50.6369) knots 0 0 0 1 2 2 2
  spline S181 degree 2 poles (9.6025, 50.6369) (10.0564, 51.0166) (11.2142, 51.4149) (12.0942, 51.4149) knots 0 0 0 1 2 2 2
  point P0 (97.4979, 0)
  constraints: 2 end point, 2 midpoint, 1 horizontal
emboss "Emboss1" sketch "Sketch3" operation cut depth 1.905 direction (0, -1, 0)
equation "\"d0\" = oneInch"
equation "\"d1\" = sevenEights"
equation "\"d2\" = drillSpacing"
equation "\"d3\" = threeQuarters"
equation "\"d5\" = drillSpacing"
equation "\"d6\" = fiveEights"
equation "\"d7\" = drillSpacing"
equation "\"d8\" = oneHalf"
equation "\"d9\" = wallSpacing"
equation "\"d10\" = wallSpacing"
equation "\"d11\" = wallSpacing"
equation "\"d12\" = wallSpacing"
equation "\"oneHalf\" = 13.335"
equation "\"fiveEights\" = 16.51"
equation "\"threeQuarters\" = 19.685"
equation "\"sevenEights\" = 22.86"
equation "\"oneInch\" = 26.035"
equation "\"drillSpacing\" = 3.175"
equation "\"wallSpacing\" = 3.175"
body "Solid1"
